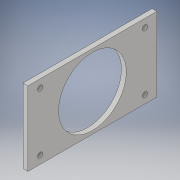
# Autodesk Inventor part: nhk30
Saved by Autodesk Inventor 2019 (Build 230136000, 136)
## iProperties
Created: 2022-02-27
Part Number: nhk30
Material: 一般
Document SubType Name: Sheet Metal
Designer: yuta
Density: 1 g/cm^3
Sheet Metal Rule: Default_mm
Appearance: 既定
Author: yuta
Autodesk Inventor part; units mm, degrees
ref_plane "YZ Plane" through (0, 0, 0) normal (1, 0, 0) x (0, 1, 0)
ref_plane "XZ Plane" through (0, 0, 0) normal (0, 1, 0) x (-1, 0, 0)
ref_plane "XY Plane" through (0, 0, 0) normal (0, 0, 1) x (1, 0, 0)
sketch "スケッチ1" plane through (0, 0, 0) normal (1, 0, 0) x (0, 1, 0)
  line L0 (0, 0) -> (46, 0)
  line L1 (46, 0) -> (46, -80)
  line L2 (46, -80) -> (0, -80)
  line L3 (0, -80) -> (0, 0)
  dimension "d0" = 46
  dimension "d1" = 80
  constraints: 8 end point, 2 parallel, 1 horizontal, 1 perpendicular
  measures "d0" distance of L1.end L2.end
  measures "d1" distance of L0.end L1.end
extrude "押し出し1" add sketch "スケッチ1" along normal blind 3
sketch "スケッチ2" plane through (3, 0, 0) normal (1, 0, 0) x (0, 0, -1)
  circle A0 centre (40, 23) radius 21
  line L0 (80, 46) -> (0, 46) projected
  line L1 (0, 46) -> (0, 0) projected
  dimension "d4" = 42
  dimension "d5" = 23
  dimension "d6" = 40
  constraints: 1 centre point
  measures "d4" diameter of A0
  measures "d5" distance from line of L0 A0.centre
  measures "d6" distance from line of L1 A0.centre
extrude "押し出し2" cut sketch "スケッチ2" against normal blind 3
sketch "スケッチ3" plane through (3, 0, 0) normal (1, 0, 0) x (0, 0, -1)
  circle A0 centre (72.5, 41) radius 1.6
  line L0 (80, 0) -> (80, 46) projected
  line L1 (80, 46) -> (0, 46) projected
  circle A1 centre (72.5, 5) radius 1.6
  line L2 (0, 0) -> (80, 0) projected
  circle A2 centre (7.5, 41) radius 1.6
  line L3 (0, 46) -> (0, 0) projected
  circle A3 centre (7.5, 5) radius 1.6
  dimension "d9" = 3.2
  dimension "d10" = 7.5
  dimension "d11" = 5
  dimension "d12" = 3.2
  dimension "d13" = 5
  dimension "d14" = 3.2
  dimension "d15" = 5
  dimension "d16" = 7.5
  dimension "d17" = 3.2
  dimension "d18" = 5
  dimension "d19" = 7.5
  dimension "d20" = 7.5
  constraints: 4 centre point
  measures "d9" diameter of A0
  measures "d10" distance from line of L0 A0.centre
  measures "d11" distance from line of L1 A0.centre
  measures "d12" diameter of A1
  measures "d13" distance from line of L2 A1.centre
  measures "d14" diameter of A2
  measures "d15" distance from line of L1 A2.centre
  measures "d16" distance from line of L3 A2.centre
  measures "d17" diameter of A3
  measures "d18" distance from line of L2 A3.centre
  measures "d19" distance from line of L3 A3.centre
  measures "d20" distance from line of L0 A1.centre
hole "穴1" at (3, 41, -7.5) at (3, 5, -7.5) at (3, 5, -72.5) at (3, 41, -72.5) direction (-1, 0, 0) diameter 3.2 depth 3
equation "\"BendRadius\" = Thickness"
equation "\"BendReliefWidth\" = Thickness"
equation "\"BendReliefDepth\" = 0.5 * Thickness"
equation "\"CornerReliefSize\" = 4 * Thickness"
equation "\"MinimumRemnant\" = 2 * Thickness"
equation "\"TransitionRadius\" = BendRadius"
equation "\"JacobiRadiusSize\" = BendRadius"
equation "\"GapSize\" = Thickness"
equation "\"Thickness\" = 0.5"
